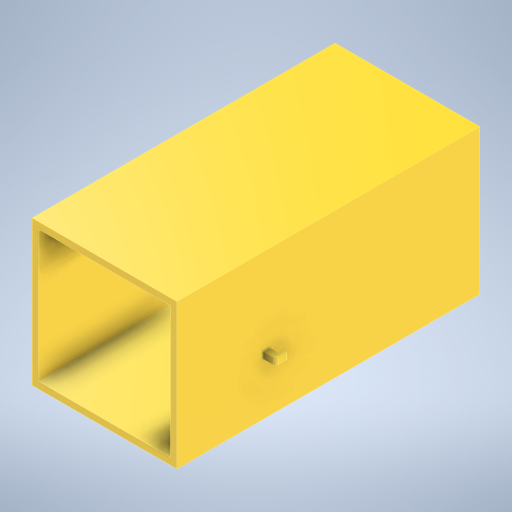
# Autodesk Inventor part: EE1
Saved by Autodesk Inventor 2024 (Build 280153000, 153)
## iProperties
Created: 2023-06-03
Part Number: EE1
Material: Glass
Document SubType Name: Modeling
Designer: raich
Density: 2.18 g/cm^3
Appearance: Glossy - Gold
Author: raich
Autodesk Inventor part; units mm, degrees
ref_plane "YZ Plane" through (0, 0, 0) normal (1, 0, 0) x (0, 1, 0)
ref_plane "XZ Plane" through (0, 0, 0) normal (0, 1, 0) x (-1, 0, 0)
ref_plane "XY Plane" through (0, 0, 0) normal (0, 0, 1) x (1, 0, 0)
sketch "Sketch1" plane through (0, 0, 0) normal (0, 0, 1) x (1, 0, 0)
  line L0 (0, -0.3318) -> (0, 109.6682)
  line L1 (0, 109.6682) -> (5, 109.6682)
  line L2 (5, 109.6682) -> (5, -0.3318)
  line L3 (5, -0.3318) -> (0, -0.3318)
  point P0 (0, 0)
  dimension "d0" = 110
  dimension "d1" = 5
  dimension "d2" = 110
  constraints: 8 end point, 2 vertical, 1 horizontal
  measures "d0" distance of L0.start L0.end
  measures "d1" distance of L0.end L1.end
  measures "d2" distance of L1.end L2.end
extrude "Extrusion1" add sketch "Sketch1" against normal blind 170
sketch "Sketch2" plane through (0, 0, 0) normal (0, 0, 1) x (1, 0, 0)
  line L0 (5, -0.3318) -> (0, -0.3318) projected
  line L1 (0, -0.3318) -> (-100, -0.3318)
  line L2 (-100, -0.3318) -> (-100, 4.6682)
  line L3 (-100, 4.6682) -> (0, 4.6682)
  point P0 (0, 0)
  dimension "d5" = 100
  dimension "d6" = 5
  dimension "d7" = 100
  constraints: 6 end point, 2 horizontal, 1 vertical
  measures "d5" distance of L0.end L1.end
  measures "d6" distance of L1.end L2.end
  measures "d7" distance of L2.end L3.end
extrude "Extrusion2" add sketch "Sketch2" against normal blind 170 fills toward (2.5, -0.2818) open curves L0 L1 L2 L3
sketch "Sketch3" plane through (0, 0, 0) normal (0, 0, 1) x (1, 0, 0)
  line L0 (-100, -0.3318) -> (5, -0.3318) projected
  line L1 (-100, -0.3318) -> (-105, -0.3318)
  line L2 (-105, -0.3318) -> (-105, 109.6682)
  line L3 (-105, 109.6682) -> (-100, 109.6682)
  line L4 (-100, 109.6682) -> (-100, -0.3318)
  point P0 (0, 0)
  dimension "d11" = 5
  dimension "d12" = 110
  dimension "d13" = 5
  constraints: 8 end point, 1 horizontal, 1 perpendicular, 1 vertical
  measures "d11" distance of L0.start L1.end
  measures "d12" distance of L1.end L2.end
  measures "d13" distance of L2.end L3.end
extrude "Extrusion3" add sketch "Sketch3" against normal blind 170
sketch "Sketch4" plane through (0, 0, 0) normal (0, 0, 1) x (1, 0, 0)
  line L0 (0, 109.6682) -> (0, 4.6682) projected
  line L1 (0, 109.6682) -> (0, 104.6682)
  line L2 (0, 104.6682) -> (-100, 104.6682)
  line L3 (-100, 4.6682) -> (-100, 109.6682) projected
  line L4 (-100, 109.6682) -> (0, 109.6682)
  point P0 (0, 0)
  dimension "d16" = 5
  dimension "d17" = 100
  dimension "d18" = 100
  constraints: 6 end point, 2 horizontal, 1 point on line
  measures "d16" distance of L0.start L1.end
  measures "d17" distance of L1.end L2.end
  measures "d18" distance of L3.end L0.start
extrude "Extrusion4" add sketch "Sketch4" against normal blind 170
sketch "Sketch5" plane through (5, -0.3318, 0) normal (1, 0, 0) x (0, 0, -1)
  line L0 (65, 45) -> (70, 45)
  line L1 (70, 45) -> (70, 40)
  line L2 (70, 40) -> (65, 40)
  line L3 (65, 40) -> (65, 45)
  point P0 (0, 0.3318)
  dimension "d21" = 5
  dimension "d22" = 5
  constraints: 8 end point, 2 parallel, 1 horizontal, 1 perpendicular
  measures "d21" distance of L1.end L2.end
  measures "d22" distance of L0.end L1.end
sketch "Sketch6" plane through (-105, -0.3318, 0) normal (-1, 0, 0) x (0, 0, 1)
  line L0 (-65, 45) -> (-70, 45)
  line L1 (-70, 45) -> (-70, 40)
  line L2 (-70, 40) -> (-65, 40)
  line L3 (-65, 40) -> (-65, 45)
  point P0 (0, 0.3318)
  dimension "d23" = 5
  dimension "d24" = 5
  constraints: 8 end point, 2 parallel, 1 horizontal, 1 perpendicular
  measures "d23" distance of L2.end L1.end
  measures "d24" distance of L1.end L0.end
extrude "Extrusion5" add sketch "Sketch5" along normal blind 10
extrude "Extrusion6" add sketch "Sketch6" along normal blind 10
fillet "Fillet1" radius 2 1 edges at (15, 42.1682, -65)
fillet "Fillet2" radius 2 1 edges at (-115, 42.1682, -65)
sketch "Sketch7" plane through (5, 39.6682, -70) normal (0, 0, -1) x (-1, 0, 0)
  line L0 (-10, 0) -> (-10, 5) projected
  line L1 (-8, 5) -> (-8, 0) projected
  line L2 (-10, 5) -> (-8, 5)
  line L3 (-8, 5) -> (-8, 0)
  line L4 (-8, 0) -> (-10, 0)
  line L5 (-10, 0) -> (-10, 5)
  line L6 (110, 5) -> (120, 5) projected
  line L7 (119.9075, 0) -> (117.9075, 0)
  line L8 (117.9075, 0) -> (117.9075, 5)
  line L9 (117.9075, 5) -> (119.9075, 5)
  line L10 (119.9075, 5) -> (119.9075, 0)
  point P0 (5, -39.6682)
  dimension "d31" = 2
  constraints: 16 end point, 4 parallel, 2 horizontal, 2 perpendicular, 2 point on line
  measures "d31" distance of L8.end L9.end
extrude "Extrusion7" add sketch "Sketch7" along normal blind 5 contours L0 L2 L1 L4
sketch "Sketch8" plane through (-105, 39.6682, -70) normal (0, 0, -1) x (-1, 0, 0)
  line L0 (0, 0) -> (10, 0) projected
  line L1 (0, 5) -> (10, 5) projected
  line L2 (10, 0) -> (8, 0)
  line L3 (8, 0) -> (8, 5)
  line L4 (8, 5) -> (10, 5)
  line L5 (10, 5) -> (10, 0)
  point P0 (-105, -39.6682)
  point P1 (8, 0)
  dimension "d34" = 2
  constraints: 8 end point, 2 parallel, 1 horizontal, 1 perpendicular, 1 point on line
  measures "d34" distance of L3.end L4.end
extrude "Extrusion8" add sketch "Sketch8" along normal blind 5
fillet "Fillet3" radius 2 2 edges at (15, 42.1682, -75) (-115, 42.1682, -75)
sketch "Sketch9" plane through (0, 0, -170) normal (0, 0, -1) x (-1, 0, 0)
  line L0 (-5, -0.3318) -> (105, -0.3318) projected
  line L1 (105, 109.6682) -> (-5, 109.6682) projected
  line L2 (-5, -0.3318) -> (105, -0.3318)
  line L3 (105, -0.3318) -> (105, 109.6682)
  line L4 (105, 109.6682) -> (-5, 109.6682)
  line L5 (-5, 109.6682) -> (-5, -0.3318)
  line L6 (100, 4.6682) -> (0, 4.6682) projected
  line L7 (0, 104.6682) -> (100, 104.6682) projected
  line L8 (0, 4.6682) -> (100, 4.6682)
  line L9 (100, 4.6682) -> (100, 104.6682)
  line L10 (100, 104.6682) -> (0, 104.6682)
  line L11 (0, 104.6682) -> (0, 4.6682)
  point P0 (0, 0)
  constraints: 16 end point, 4 parallel, 2 horizontal, 2 perpendicular
extrude "Extrusion9" add sketch "Sketch9" along normal blind 60
body "Solid1"
